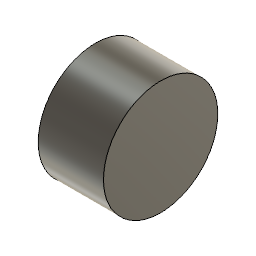
Rc Car (Autodesk Fusion 360 archive; units mm, degrees)
design "Wheels"
part number: 2026-03-18-11-04-32-941
Autodesk Fusion 360 part; units mm, degrees
sketch "Sketch1" plane through (0, 0, 0) normal (1, 0, 0) x (0, 1, 0)
  circle A0 centre (0, 0) radius 35
  dimension "d1" = 70
  constraint coincident A0.centre origin
  measures "d1" diameter of A0
extrude "Extrude1" add sketch "Sketch1" along normal blind 40

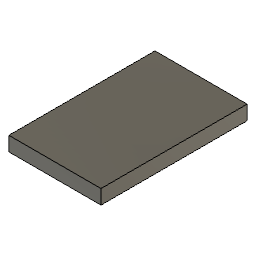
design "breadboard 400 pin"
part number: 2026-03-18-11-13-13-110
Autodesk Fusion 360 part; units mm, degrees
sketch "Sketch1" plane through (0, 0, 0) normal (0, 0, 1) x (1, 0, 0)
  line L0 (26.5, -42) -> (-26.5, -42)
  line L1 (-26.5, -42) -> (-26.5, 42)
  line L2 (-26.5, 42) -> (26.5, 42)
  line L3 (26.5, 42) -> (26.5, -42)
  line L4 (26.5, -42) -> (-26.5, 42) construction
  line L5 (-26.5, -42) -> (26.5, 42) construction
  dimension "d1" = 53
  dimension "d2" = 84
  constraint horizontal L0
  constraint perpendicular L0 L1
  constraint parallel L0 L2
  constraint parallel L1 L3
  constraint coincident L4 origin
  constraint coincident L5 origin
  measures "d1" distance of L1.end L2.end
  measures "d2" distance of L0.end L1.end
extrude "Extrude1" add sketch "Sketch1" along normal blind 8.3
